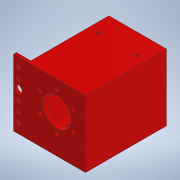
# Autodesk Inventor part: ViperSlide Motor Mount
Saved by Autodesk Inventor 2022 (Build 260153000, 153)
## iProperties
Created: 2022-09-17
Part Number: ViperSlide Motor Mount
Material: Generic
Document SubType Name: Modeling
Designer: matt
Density: 1 g/cm^3
Appearance: Default
Author: matt
Autodesk Inventor part; units mm, degrees
ref_plane "YZ Plane" through (0, 0, 0) normal (1, 0, 0) x (0, 1, 0)
sketch "Sketch1" plane through (0, 0, 0) normal (0, 0, 1) x (1, 0, 0)
  circle A0 centre (36, 40) radius 1.7
  line L0 (0, 0) -> (12, 0)
  line L1 (0, 0) -> (0, 384)
  line L2 (12, 384) -> (12, -8)
  circle A1 centre (4, 8) radius 2
  circle A2 centre (36, 24) radius 12
  line L3 (0, 0) -> (60, 0)
  line L4 (60, 0) -> (60, 47.4892)
  line L5 (60, 46) -> (0, 46)
  line L6 (0, 46) -> (0, 0)
  line L7 (0, 4) -> (60, 4)
  circle A3 centre (22.1436, 32) radius 1.7
  circle A4 centre (22.1436, 16) radius 1.7
  circle A5 centre (36, 8) radius 1.7
  circle A6 centre (49.8564, 16) radius 1.7
  circle A7 centre (49.8564, 32) radius 1.7
  circle A8 centre (4, 16) radius 2
  circle A9 centre (4, 24) radius 2
  circle A10 centre (4, 32) radius 2
  circle A11 centre (4, 40) radius 2
  line L8 (22.731, 4) -> (14.2875, 18.6246)
  line L9 (14.2875, 18.6246) -> (12, 18.6246)
  line L10 (36, 0) -> (36, 40) construction
  line L11 (49.269, 4) -> (57.7125, 18.6246)
  line L12 (57.7125, 18.6246) -> (60, 18.6246)
  line L13 (60, 23.7446) -> (12, 23.7446) construction
  line L14 (0, 47.4892) -> (60, 47.4892)
  line L15 (22.731, 43.4892) -> (14.2875, 28.8646)
  line L16 (14.2875, 28.8646) -> (12, 28.8646)
  line L17 (57.7125, 28.8646) -> (60, 28.8646)
  line L18 (49.269, 43.4892) -> (57.7125, 28.8646)
  line L19 (0, 43.4892) -> (12, 43.4892)
  line L20 (22.731, 43.4892) -> (49.269, 43.4892)
  line L21 (60, 28.8646) -> (58.8562, 28.8646)
  line L22 (58.8562, 28.8646) -> (58.8562, 18.6246)
  line L23 (58.8562, 18.6246) -> (60, 18.6246)
  line L24 (60, 18.6246) -> (60, 28.8646)
  line L25 (13.1437, 28.8646) -> (13.1437, 18.6246)
  circle A12 centre (4, 24) radius 3.25
  line L26 (0, 0) -> (60, 0)
  line L27 (60, 0) -> (60, -8)
  line L28 (60, -8) -> (0, -8)
  line L29 (0, -8) -> (0, 0)
  line L30 (0, -4) -> (60, -4)
  circle A13 centre (4, 0) radius 2
  line L31 (41.275, 0) -> (30, 0)
  line L32 (30, 4) -> (30, -4)
  line L33 (30, -4) -> (41.275, -4)
  line L34 (41.275, -4) -> (41.275, 4)
  circle A14 centre (4, 16) radius 3.25
  point P0 (12, 46)
  point P1 (12, 0)
  point P2 (12, 4)
  point P3 (0, 47.4892)
  point P4 (60, 43.4892)
  point P5 (12, 47.4892)
  point P6 (2, 0)
  point P7 (6, 0)
  dimension "d1" = 3.4
  dimension "d2" = 24
  dimension "d7" = 4
  dimension "d8" = 46
  dimension "d9" = 24
  dimension "d10" = 16
  dimension "d13" = 360
  dimension "d15" = 8
  dimension "d16" = 4
  dimension "d17" = 8
  dimension "d20" = 8
  dimension "d34" = 6.5
  dimension "d35" = 8
  dimension "d36" = 4
  dimension "d39" = 6.5
  constraints: 70 end point, 17 point on line, 15 centre point, 15 symmetric about line, 8 parallel, 7 midpoint, 7 perpendicular, 4 horizontal, 2 coincident, 1 vertical, 21 other
  measures "d1" diameter of A0
  measures "d2" diameter of A2
  measures "d7" distance between parallel lines of L3 L7
  measures "d8" distance between parallel lines of L3 L5
  measures "d9" distance from line of L3 A2.centre
  measures "d10" distance of A2.centre L10.end
  measures "d15" distance from line of L0 A1.centre
  measures "d16" diameter of A1
  measures "d17" distance from line of L2 A1.centre
  measures "d20" distance of A1.centre A8.centre
  measures "d34" diameter of A12
  measures "d35" distance between parallel lines of L28 L3
  measures "d36" diameter of A13
  measures "d39" diameter of A14
extrude "Extrusion1" add sketch "Sketch1" along normal blind 2.5 contours A13 L0 L1 L7 L2 | A13 L0 | L0 A13 | L0 L2 L30 L29 A13 | L3 L32 L30 L2 | L2 L7 L32 L3 | L7 L1 L19 L2 | L2 L9 L8 L7 | L30 L27 L28 L2 | L2 L28 L29 L30 | L32 L7 L34 L3 | L3 L34 L30 L32 | L2 L16 L25 L9 | L8 L9 L25 L16 L15 L20 L18 L17 L22 L12 L11 L7 | L34 L7 L4 L3 | L3 L27 L30 L34 | L2 L5 L4 L17 L18 L20 L15 L16 | L1 L5 L2 L19 | L1 L14 L2 L5 | L7 L11 L12 L4 | L2 L14 L4 L5 | L12 L22 L17 L4 | A8 | A10 | A14
extrude "Extrusion2" add sketch "Sketch1" against normal blind 2 contours L3 L32 L30 L2 | L2 L7 L32 L3 | L2 L9 L8 L7 | L30 L27 L28 L2 | L32 L7 L34 L3 | L3 L34 L30 L32 | L2 L16 L25 L9 | L8 L9 L25 L16 L15 L20 L18 L17 L22 L12 L11 L7 | L34 L7 L4 L3 | L3 L27 L30 L34 | L2 L5 L4 L17 L18 L20 L15 L16 | L7 L11 L12 L4 | L2 L14 L4 L5 | L12 L22 L17 L4
extrude "Extrusion3" add sketch "Sketch1" against normal blind 65 contours L3 L32 L30 L2 | L2 L7 L32 L3 | L2 L9 L8 L7 | L30 L27 L28 L2 | L3 L34 L30 L32 | L2 L16 L25 L9 | L34 L7 L4 L3 | L3 L27 L30 L34 | L2 L5 L4 L17 L18 L20 L15 L16 | L7 L11 L12 L4 | L2 L14 L4 L5 | L12 L22 L17 L4
sketch "Sketch2" plane through (22.731, 4, -2) normal (0, 1, 0) x (1, 0, 0)
  line L0 (26.5379, 0) -> (0, 0) construction
  line L1 (13.269, 0) -> (12.9065, 63) construction
  line L2 (7.269, 63) -> (18.544, 63) construction
  circle A0 centre (13.1798, 15.5) radius 2.8
  circle A1 centre (12.9957, 47.4995) radius 2.8
  circle A2 centre (29.269, 46.0997) radius 1.55
  circle A3 centre (-2.731, 46.0997) radius 1.55
  point P0 (-22.731, -2)
  point P1 (37.269, 50)
  point P2 (-10.731, 50)
  dimension "d27" = 5.6
  dimension "d28" = 5.6
  dimension "d29" = 32
  dimension "d30" = 63
  dimension "d31" = 15.5
  dimension "d40" = 3.1
  dimension "d41" = 3.1
  constraints: 4 centre point, 2 end point, 2 point on line, 1 midpoint, 2 other
  measures "d27" diameter of A0
  measures "d28" diameter of A1
  measures "d29" distance of A1.centre A0.centre
  measures "d31" distance from line of A0.centre L0
  measures "d40" diameter of A2
  measures "d41" diameter of A3
extrude "Extrusion5" cut sketch "Sketch2" against normal blind 52 contours A0 | A1
extrude "Extrusion6" cut sketch "Sketch2" against normal blind 12 from surface at 43.4892 contours A2 | A3
ref_plane "Work Plane1" through (0, -8, -48) normal (0, 0, -1) x (0, 1, 0)
extrude "Extrusion7" add sketch "Sketch1" against normal blind 4 from surface at -48 contours A13 L0 L1 L7 L2 | A13 L0 | L0 A13 | L0 L2 L30 L29 A13 | L7 L1 L19 L2 | L2 L28 L29 L30 | L1 L5 L2 L19 | L1 L14 L2 L5 | A8 | A10 | A12 | A14
ref_plane "Work Plane2" through (0, -8, -48) normal (0, 0, -1) x (0, 1, 0)
extrude "Extrusion8" cut sketch "Sketch1" against normal blind 0.5 from surface at -48 contours A13 L0 L1 L7 L2 | A13 L0 | L0 A13 | L0 L2 L30 L29 A13 | L7 L1 L19 L2 | L2 L28 L29 L30 | L1 L5 L2 L19 | L1 L14 L2 L5 | A8 | A10 | A12 | A14
equation "\"d31\" = -0.5 * d29 + 0.5 * d30"
equation "\"d41\" = d40"
body "Solid1"
